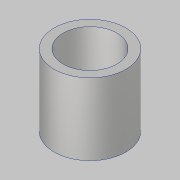
# Autodesk Inventor part: PlaceholderSmall
Saved by Autodesk Inventor 2019.2 (Build 232265000, 265)
## iProperties
Created: 2019-02-06
Part Number: PlaceholderSmall
Material: Aluminium 6061
Document SubType Name: Modeling
Designer: Lion
Density: 2.7 g/cm^3
Appearance: Aluminium - flach
Author: Lion
Autodesk Inventor part; units mm, degrees
ref_plane "YZ Plane" through (0, 0, 0) normal (1, 0, 0) x (0, 1, 0)
ref_plane "XZ Plane" through (0, 0, 0) normal (0, 1, 0) x (-1, 0, 0)
ref_plane "XY Plane" through (0, 0, 0) normal (0, 0, 1) x (1, 0, 0)
sketch "Skizze1" plane through (0, 0, 0) normal (0, 1, 0) x (-1, 0, 0)
  circle A0 centre (0, 0) radius 1.5
  circle A1 centre (0, 0) radius 2
  dimension "d1" = 0.5
  dimension "d2" = 4
  constraints: 2 centre point, 2 coincident
  measures "d1" radial gap between concentric circles of A1 A0
  measures "d2" diameter of A1
extrude "Extrusion1" add sketch "Skizze1" along normal blind 4
